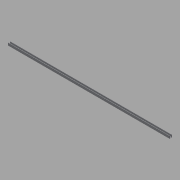
# Autodesk Inventor part: 26in mini C-Channel (rail)
Saved by Autodesk Inventor 2013 (Build 170138000, 138)
## iProperties
Created: 2013-01-27
Part Number: 26in mini C-Channel (rail)
Material: Aluminum 6061
Document SubType Name: Modeling
Designer: Naphat
Density: 1 g/cm^3
Author: Naphat
Autodesk Inventor part; units mm, degrees
ref_plane "YZ Plane" through (0, 0, 0) normal (1, 0, 0) x (0, 1, 0)
ref_plane "XZ Plane" through (0, 0, 0) normal (0, 1, 0) x (-1, 0, 0)
ref_plane "XY Plane" through (0, 0, 0) normal (0, 0, 1) x (1, 0, 0)
sketch "Sketch1" plane through (0, 0, 0) normal (1, 0, 0) x (0, 1, 0)
  line L0 (0, 0) -> (0, -10)
  line L1 (0, -10) -> (10, -10)
  line L2 (10, -10) -> (10, -8.5)
  line L3 (0, 0) -> (10, 0)
  line L4 (10, 0) -> (10, -1.5)
  line L5 (0, -5) -> (1.5, -5) construction
  line L6 (10, -1.5) -> (1.5, -1.5)
  line L7 (1.5, -1.5) -> (1.5, -8.5)
  line L8 (1.5, -8.5) -> (10, -8.5)
  dimension "d0" = 10
  dimension "d1" = 10
  dimension "d2" = 1.5
  dimension "d3" = 10
  dimension "d4" = 1.5
  dimension "d5" = 1.5
  constraints: 18 end point, 5 perpendicular, 3 parallel, 1 midpoint, 1 vertical
  measures "d0" distance of L0.start L0.end
  measures "d1" distance of L0.end L1.end
  measures "d2" distance of L1.end L2.end
  measures "d3" distance of L0.start L3.end
  measures "d4" distance of L3.end L4.end
  measures "d5" distance of L5.start L5.end
extrude "Extrusion1" add sketch "Sketch1" along normal blind 660.4
body "Solid1"
